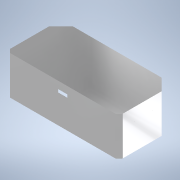
# Autodesk Inventor part: Carcasa
Saved by Autodesk Inventor 2022.1 (Build 261234000, 234)
## iProperties
Created: 2021-10-13
Part Number: Carcasa
Material: Aluminio 6061
Document SubType Name: Sheet Metal
Designer: seb_0
Density: 2.7 g/cm^3
Appearance: Aluminio - Plano
Sheet Metal Rule: Por defecto_mm
Author: seb_0
Autodesk Inventor part; units mm, degrees
ref_plane "YZ Plane" through (0, 0, 0) normal (1, 0, 0) x (0, 1, 0)
ref_plane "XZ Plane" through (0, 0, 0) normal (0, 1, 0) x (-1, 0, 0)
ref_plane "Plano de trabajo1" through (0, 15.93, 0) normal (0, 0, 1) x (1, 0, 0)
sketch "Boceto1" plane through (0, 15.93, 0) normal (0, 0, 1) x (1, 0, 0)
  line L0 (225, 372.2908) -> (225, -4.1508) projected
  line L1 (224.6622, -4.9663) -> (193.0363, -36.5922) projected
  line L2 (113.0363, 484.7322) -> (224.6622, 373.1063) projected
  line L3 (-744.2208, 485.07) -> (112.2208, 485.07) projected
  line L4 (-857, -4.1508) -> (-857, 372.2908) projected
  line L5 (-825.0363, -36.5922) -> (-856.6622, -4.9663) projected
  line L6 (-856.6622, 373.1063) -> (-745.0363, 484.7322) projected
  line L7 (224.6622, 373.1063) -> (225, 372.2908)
  line L8 (112.2208, 485.07) -> (113.0363, 484.7322)
  line L9 (225, -4.1508) -> (224.6622, -4.9663)
  line L10 (192.2208, -36.93) -> (-824.2208, -36.93) projected
  line L11 (192.2208, -36.93) -> (193.0363, -36.5922)
  line L12 (-825.0363, -36.5922) -> (-824.2208, -36.93)
  line L13 (-857, -4.1508) -> (-856.6622, -4.9663)
  line L14 (-857, 372.2908) -> (-856.6622, 373.1063)
  line L15 (-745.0363, 484.7322) -> (-744.2208, 485.07)
  line L16 (-858.5, -4.4491) -> (-860.9339, 1.4267)
  line L17 (-824.5191, -38.43) -> (192.5191, -38.43)
  line L18 (192.5191, -38.43) -> (193.886, -37.8639)
  line L19 (193.886, -37.8639) -> (225.9339, -5.816)
  line L20 (225.9339, -5.816) -> (226.5, -4.4491)
  line L21 (226.5, -4.4491) -> (226.5, 372.5891)
  line L22 (226.5, 372.5891) -> (225.9339, 373.956)
  line L23 (225.9339, 373.956) -> (113.886, 486.0039)
  line L24 (113.886, 486.0039) -> (112.5191, 486.57)
  line L25 (112.5191, 486.57) -> (-744.5191, 486.57)
  line L26 (-744.5191, 486.57) -> (-745.886, 486.0039)
  line L27 (-745.886, 486.0039) -> (-857.9339, 373.956)
  line L28 (-857.9339, 373.956) -> (-858.5, 372.5891)
  line L29 (-858.5, 372.5891) -> (-858.5, -4.4491)
  line L30 (-858.5, -4.4491) -> (-857.9339, -5.816)
  line L31 (-857.9339, -5.816) -> (-825.886, -37.8639)
  line L32 (-825.886, -37.8639) -> (-824.5191, -38.43)
  point P0 (0, -15.93)
  dimension "d63" = 1.5
  constraints: 50 end point, 8 perpendicular, 15 other
  measures "d63" distance between parallel lines of L10 L17
extrude "Extrusión1" add sketch "Boceto1" against normal blind 371.581
sketch "Boceto2" plane through (0, 15.93, 0) normal (0, 0, 1) x (1, 0, 0)
  line L0 (-857, -4.1508) -> (-857, 372.2908)
  line L1 (-857, 372.2908) -> (-856.6622, 373.1063)
  line L2 (-856.6622, 373.1063) -> (-745.0363, 484.7322)
  line L3 (-745.0363, 484.7322) -> (-744.2208, 485.07)
  line L4 (-744.2208, 485.07) -> (112.2208, 485.07)
  line L5 (112.2208, 485.07) -> (113.0363, 484.7322)
  line L6 (113.0363, 484.7322) -> (224.6622, 373.1063)
  line L7 (224.6622, 373.1063) -> (225, 372.2908)
  line L8 (225, 372.2908) -> (225, -4.1508)
  line L9 (225, -4.1508) -> (224.6622, -4.9663)
  line L10 (224.6622, -4.9663) -> (193.0363, -36.5922)
  line L11 (-825.0363, -36.5922) -> (-856.6622, -4.9663)
  line L12 (-825.0363, -36.5922) -> (-856.6622, -4.9663)
  line L13 (224.6622, -4.9663) -> (193.0363, -36.5922)
  line L14 (192.2208, -36.93) -> (-824.2208, -36.93)
  line L15 (-857, -4.1508) -> (-857, 372.2908)
  line L16 (193.0363, -36.5922) -> (192.2208, -36.93)
  line L17 (192.2208, -36.93) -> (-824.2208, -36.93)
  line L18 (-824.2208, -36.93) -> (-825.0363, -36.5922)
  line L19 (-825.0363, -36.5922) -> (-856.6622, -4.9663)
  line L20 (-856.6622, -4.9663) -> (-857, -4.1508)
  line L21 (112.5191, 486.57) -> (-744.5191, 486.57)
  line L22 (-825.886, -37.8639) -> (-824.5191, -38.43)
  line L23 (-824.5191, -38.43) -> (192.5191, -38.43)
  line L24 (192.5191, -38.43) -> (193.886, -37.8639)
  line L25 (193.886, -37.8639) -> (225.9339, -5.816)
  line L26 (225.9339, -5.816) -> (226.5, -4.4491)
  line L27 (226.5, -4.4491) -> (226.5, 372.5891)
  line L28 (226.5, 372.5891) -> (225.9339, 373.956)
  line L29 (225.9339, 373.956) -> (113.886, 486.0039)
  line L30 (113.886, 486.0039) -> (112.5191, 486.57)
  line L31 (112.5191, 486.57) -> (-744.5191, 486.57)
  line L32 (-744.5191, 486.57) -> (-745.886, 486.0039)
  line L33 (-745.886, 486.0039) -> (-857.9339, 373.956)
  line L34 (-857.9339, 373.956) -> (-858.5, 372.5891)
  line L35 (-858.5, 372.5891) -> (-858.5, -4.4491)
  line L36 (-858.5, -4.4491) -> (-857.9339, -5.816)
  line L37 (-857.9339, -5.816) -> (-825.886, -37.8639)
  line L38 (-857, -4.1508) -> (-857, 372.2908)
  line L39 (-857, 372.2908) -> (-856.6622, 373.1063)
  line L40 (-856.6622, 373.1063) -> (-745.0363, 484.7322)
  line L41 (-745.0363, 484.7322) -> (-744.2208, 485.07)
  line L42 (-744.2208, 485.07) -> (112.2208, 485.07)
  line L43 (112.2208, 485.07) -> (113.0363, 484.7322)
  line L44 (113.0363, 484.7322) -> (224.6622, 373.1063)
  line L45 (224.6622, 373.1063) -> (225, 372.2908)
  line L46 (225, 372.2908) -> (225, -4.1508)
  line L47 (225, -4.1508) -> (224.6622, -4.9663)
  line L48 (224.6622, -4.9663) -> (193.0363, -36.5922)
  line L49 (193.0363, -36.5922) -> (192.2208, -36.93)
  line L50 (192.2208, -36.93) -> (-824.2208, -36.93)
  line L51 (-824.2208, -36.93) -> (-825.0363, -36.5922)
  line L52 (-825.0363, -36.5922) -> (-856.6622, -4.9663)
  line L53 (-856.6622, -4.9663) -> (-857, -4.1508)
  point P0 (-824.2208, -36.93)
extrude "Extrusión2" add sketch "Boceto2" along normal blind 1.5 contours L0 L1 L2 L3 L4 L5 L6 L7 L8 L9 L10 L16 L14 L18 L11 L20 | L30 L29 L28 L27 L26 L25 L24 L23 L22 L37 L36 L35 L34 L33 L32 L21
sketch "Boceto4" plane through (-744.5191, 502.5, -371.581) normal (0, 1, 0) x (1, 0, 0)
  line L0 (855.1466, -300) -> (1.8917, -300) projected
  circle A0 centre (655.1466, -280) radius 2.5
  circle A1 centre (201.8917, -251.581) radius 2.5
  line L1 (857.0383, -373.081) -> (0, -373.081) projected
  point P0 (744.5191, -371.581)
  dimension "d7" = 5
  dimension "d8" = 200
  dimension "d9" = 200
  dimension "d86" = 20
  dimension "d87" = 121.5
  constraints: 2 centre point, 1 equal radius
  measures "d7" diameter of A0
  measures "d8" horizontal distance of L0.start A0.centre
  measures "d9" horizontal distance of A1.centre L0.end
  measures "d86" distance from line of L0 A0.centre
  measures "d87" distance from line of L1 A1.centre
hole "Agujero1" at (-89.3726, 502.5, -91.581) at (-542.6274, 502.5, -120) direction (0, -1, 0) diameter 2.459 depth 8.8 tip angle 118 thread size "M3x0.5" class "6H" standard "ISO Metric profile"
sketch "Boceto7" plane through (-858.5, 27.4109, -371.581) normal (-1, 0, 0) x (0, 0, 1)
  line L0 (264, 376.8034) -> (264, 0.2349) projected
  circle A0 centre (251.581, 276.8034) radius 2.5
  circle A1 centre (251.581, 100.2349) radius 2.5
  line L1 (300, 359.2166) -> (300, -14.0383) projected
  line L2 (373.081, 361.1083) -> (373.081, -15.93) projected
  point P0 (371.581, -27.4109)
  dimension "d21" = 5
  dimension "d23" = 100
  dimension "d24" = 100
  dimension "d88" = 121.5
  dimension "d89" = 121.5
  constraints: 2 centre point, 1 equal radius
  measures "d21" diameter of A0
  measures "d23" vertical distance of L0.start A0.centre
  measures "d24" vertical distance of L0.end A1.centre
  measures "d88" distance from line of L2 A0.centre
  measures "d89" distance from line of L2 A1.centre
hole "Agujero2" at (-858.5, 304.2143, -120) at (-858.5, 127.6457, -120) direction (1, 0, 0) diameter 2.459 end through all thread size "M3x0.5" class "6H" standard "ANSI Metric M Profile"
sketch "Boceto16" plane through (-744.5191, 502.5, -371.581) normal (0, 1, 0) x (1, 0, 0)
  line L0 (468.5191, -271.581) -> (468.5191, -351.581)
  line L1 (468.5191, -351.581) -> (388.5191, -351.581)
  line L2 (388.5191, -351.581) -> (388.5191, -271.581)
  line L3 (80, -271.581) -> (80, -351.581)
  line L4 (80, -351.581) -> (0, -351.581)
  line L5 (776.7399, -271.581) -> (776.7399, -351.581)
  line L6 (0, 0) -> (0, -373.081) projected
  line L7 (776.7399, -351.581) -> (856.7399, -351.581)
  line L8 (0, -351.581) -> (0, -271.581)
  line L9 (-1.3668, 0) -> (-1.3668, -373.081) projected
  line L10 (856.7399, -371.581) -> (856.7399, 0) projected
  line L11 (0, -271.581) -> (80, -271.581)
  line L12 (776.7399, -271.581) -> (856.7399, -271.581)
  line L13 (856.7399, -271.581) -> (856.7399, -351.581)
  line L14 (468.5191, -271.581) -> (388.5191, -271.581)
  line L15 (855.1466, -271.581) -> (1.8917, -271.581)
  point P0 (744.5191, -371.581)
  point P1 (468.5191, -311.581)
  point P2 (428.5191, -271.581)
  point P3 (816.7399, -271.581)
  dimension "d65" = 80
  dimension "d69" = 80
  dimension "d70" = 80
  dimension "d90" = 80
  dimension "d92" = 308.2208
  dimension "d93" = 308.5192
  constraints: 26 end point, 5 horizontal, 5 point on line, 4 midpoint, 3 perpendicular, 2 equal length, 2 vertical, 1 parallel, 2 other
  measures "d65" distance of L3.start L3.end
  measures "d69" distance of L0.end L1.end
  measures "d70" distance of L3.end L4.end
  measures "d90" distance of L5.start L5.end
  measures "d92" distance between parallel lines of L5 L0
  measures "d93" distance between parallel lines of L3 L2
sketch "Boceto17" plane through (-824.5191, -22.5, -371.581) normal (0, -1, 0) x (1, 0, 0)
  line L0 (468.5191, 303.081) -> (548.5191, 303.081)
  line L1 (553.5191, 298.081) -> (553.5191, 278.081)
  line L2 (548.5191, 273.081) -> (468.5191, 273.081)
  line L3 (463.5191, 278.081) -> (463.5191, 298.081)
  line L4 (0, 373.081) -> (1017.0383, 373.081) projected
  line L5 (463.5191, 288.081) -> (0.2984, 288.081)
  line L6 (0.2984, 371.581) -> (0.2984, 0) projected
  line L7 (553.5191, 288.081) -> (1016.7399, 288.081)
  line L8 (1016.7399, 371.581) -> (1016.7399, 0) projected
  arc A0 (468.5191, 303.081) -> (463.5191, 298.081) centre (468.5191, 298.081) ccw
  arc A1 (463.5191, 278.081) -> (468.5191, 273.081) centre (468.5191, 278.081) ccw
  arc A2 (548.5191, 273.081) -> (553.5191, 278.081) centre (548.5191, 278.081) ccw
  arc A3 (553.5191, 298.081) -> (548.5191, 303.081) centre (548.5191, 298.081) ccw
  point P0 (824.5191, 371.581)
  point P1 (463.5191, 303.081)
  point P2 (553.5191, 273.081)
  point P3 (553.5191, 303.081)
  point P4 (463.5191, 273.081)
  dimension "d71" = 70
  dimension "d72" = 30
  dimension "d73" = 90
  dimension "d76" = 5
  dimension "d77" = 5
  dimension "d78" = 5
  dimension "d79" = 5
  constraints: 12 end point, 10 point on line, 8 point on circle, 8 tangent, 4 centre point, 3 horizontal, 2 midpoint, 2 parallel, 1 collinear, 1 perpendicular
  measures "d71" distance between parallel lines of L4 L0
  measures "d72" distance of point (553.519, 303.081) point (553.519, 273.081)
  measures "d73" distance of point (463.519, 303.081) point (553.519, 303.081)
  measures "d76" radius of A0
  measures "d77" radius of A1
  measures "d78" radius of A2
  measures "d79" radius of A3
extrude "Cortar1" cut sketch "Boceto16" against normal blind 1.5
extrude "Cortar2" cut sketch "Boceto17" against normal blind 1.5
equation "\"d81\" = Grosor"
equation "\"d83\" = Grosor"
equation "\"Radio_pliegue\" = Grosor"
equation "\"Anchura_desahogo_plegado\" = Grosor"
equation "\"Profundidad_desahogo_plegado\" = 0.5 * Grosor"
equation "\"Tamaño_destalonado\" = 4 * Grosor"
equation "\"Remanente_mínimo\" = 2 * Grosor"
equation "\"Radiodetransición\" = Radio_pliegue"
equation "\"Tamaño_de_radio_de_Jacobi\" = Radio_pliegue"
equation "\"TamañoSeparación\" = Grosor"
equation "\"d80\" = Grosor"
equation "\"Grosor\" = 1.5"
